Autodesk Inventor part; units mm, degrees
(part 2 of 2)
extrude "Extrusion98" add sketch "Sketch107" against normal blind 10
sketch "Sketch108" plane through (0, 0, 50) normal (0, 0, 1) x (1, 0, 0)
  line L0 (11, -49.7965) -> (28.75, -49.7965) projected
  line L1 (11, 49.7965) -> (28.75, 49.7965) projected
  line L2 (11, -49.7965) -> (12, -49.7965)
  line L3 (12, -49.7965) -> (12, 49.7965)
  line L4 (12, 49.7965) -> (11, 49.7965)
  line L5 (11, 49.7965) -> (11, -49.7965)
  point P0 (0, 0)
  dimension "d436" = 1
  constraints: 8 end point, 2 parallel, 1 horizontal, 1 perpendicular, 1 point on line
  measures "d436" distance between parallel lines of L3 L5
extrude "Extrusion99" cut sketch "Sketch108" along normal through all
body "Solid2"
